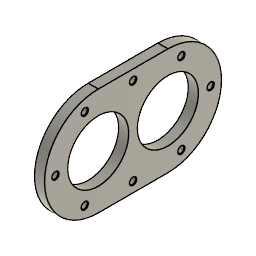
Side Plate_ (Autodesk Fusion 360 design; units mm, degrees)
Autodesk Fusion 360 part; units mm, degrees
sketch "Sketch1" plane through (0, 0, 0) normal (1, 0, 0) x (0, 1, 0)
  line L0 (24, 37) -> (-24, 37)
  arc A0 (-24, 37) -> (-24, -37) centre (-24, 0) ccw
  line L1 (-24, -37) -> (24, -37)
  arc A1 (24, -37) -> (24, 37) centre (24, 0) ccw
  line L2 (24, 0) -> (-24, 0) construction
  circle A2 centre (-24, 0) radius 21
  circle A3 centre (24, 0) radius 21
  dimension "d1" = 48
  dimension "d2" = 37
  dimension "d3" = 42
  dimension "d4" = 42
  constraint tangent L0 A0
  constraint tangent A0 L1
  constraint parallel L0 L1
  constraint tangent L1 A1
  constraint tangent L0 A1
  constraint horizontal L2
  constraint midpoint L2 origin
  constraint concentric A0 A2
  constraint concentric A1 A3
  measures "d1" distance of A1.centre A0.centre
  measures "d2" radius of A0
  measures "d3" diameter of A2
  measures "d4" diameter of A3
extrude "Extrude1" add sketch "Sketch1" along normal blind 7
sketch "Sketch2" plane through (7, 0, 0) normal (1, 0, 0) x (0, 1, 0)
  circle A0 centre (-24, 0) radius 21
  circle A1 centre (24, 0) radius 21
  arc A2 (24, -37) -> (24, 37) centre (24, 0) ccw
  line L0 (24, 37) -> (-24, 37)
  arc A3 (-24, 37) -> (-24, -37) centre (-24, 0) ccw
  line L1 (-24, -37) -> (24, -37)
  circle A4 centre (-24, 0) radius 29.5 construction
  line L2 (0, 0) -> (0, 48.4021) construction
  point P0 (0, 30)
  point P1 (-33.2871, 28)
  point P2 (-53.5, 0)
  point P3 (-33.2871, -28)
  point P4 (0, -30)
  point P5 (33.2871, 28)
  point P6 (53.5, 0)
  point P7 (33.2871, -28)
  dimension "d7" = 59
  dimension "d8" = 28
  dimension "d9" = 30
  dimension "d10" = 30
  constraint concentric A0 A4
  constraint coincident L2.start origin
  constraint vertical L2
  constraint coincident L2 P0
  constraint coincident A4 P1
  constraint coincident A4 P2
  constraint coincident A4 P3
  constraint vertical L2.start P4
  constraint horizontal A0.centre P2
  constraint vertical P1 P3
  constraint symmetric L2 P1 P5
  constraint symmetric L2 P2 P6
  constraint symmetric L2 P3 P7
  measures "d7" diameter of A4
  measures "d8" vertical distance of A0.centre P1
  measures "d9" distance of L2.start P0
  measures "d10" distance of L2.start P4
hole "Hole1" at (7, -33.2871, 28) at (7, -53.5, 0) at (7, -33.2871, -28) at (7, 0, -30) at (7, 33.2871, -28) at (7, 53.5, 0) at (7, 33.2871, 28) at (7, 0, 30) direction (-1, 0, 0) diameter 4.2 end through all countersink diameter 5 countersink angle 90
